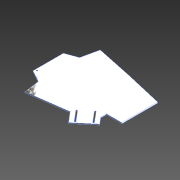
# Autodesk Inventor part: baseframe
Saved by Autodesk Inventor 2018 (Build 220112000, 112)
## iProperties
Created: 2018-05-27
Part Number: baseframe
Material: アルミニウム 6061
Document SubType Name: Sheet Metal
Designer: NaMACHAN
Mass: 118.519 g
Surface Area: 451.786 cm^2
Volume: 43.8959 cm^3
Density: 2.7 g/cm^3
Sheet Metal Rule: Default
Appearance: アルミニウム - フラット
Author: NaMACHAN
Autodesk Inventor part; units mm, degrees
ref_plane "YZ Plane" through (0, 0, 0) normal (1, 0, 0) x (0, 1, 0)
ref_plane "XZ Plane" through (0, 0, 0) normal (0, 1, 0) x (-1, 0, 0)
ref_plane "XY Plane" through (0, 0, 0) normal (0, 0, 1) x (1, 0, 0)
sketch "スケッチ1" plane through (0, 0, 0) normal (0, 0, 1) x (1, 0, 0)
  line L0 (-106.8804, 63.2098) -> (-114.8803, 63.2581) projected
  line L1 (-107.2922, -5.024) -> (-115.292, -4.9758) projected
  line L2 (-4.6996, 92.8548) -> (1.3002, 92.8186) projected
  line L3 (-5.3383, -12.9733) -> (0.6616, -13.0095) projected
  line L4 (-79.7382, 110.3105) -> (1.3027, 93.2276) projected
  line L5 (-88.2817, 72.7187) -> (-79.7382, 110.3105) projected
  line L6 (-84.055, -53.4485) -> (5.2045, -41.9275)
  line L7 (49.6711, -27.8017) -> (49.6711, -11.6868)
  line L8 (49.6711, -11.6868) -> (84.6711, -11.6868)
  line L9 (5.2045, -41.9275) -> (20.2045, -67.9083)
  line L10 (20.2045, -67.9083) -> (59.6711, -45.1223)
  line L11 (59.6711, -45.1223) -> (49.6711, -27.8017)
  line L12 (-84.055, -53.4485) -> (-90.292, -5.1266)
  circle A0 centre (-111.2619, 0) radius 1.5 projected
  circle A1 centre (-110.9105, 58.2341) radius 1.5 projected
  line L13 (-115.292, -4.9758) -> (-114.8803, 63.2581) projected
  line L14 (-106.8804, 63.2098) -> (-114.8803, 63.2581) projected
  line L15 (-106.8804, 63.2098) -> (-107.2922, -5.024) projected
  line L16 (-107.2922, -5.024) -> (-115.292, -4.9758) projected
  line L17 (-90.292, -5.1266) -> (-115.292, -4.9758)
  line L18 (-115.292, -4.9758) -> (-114.8803, 63.2581)
  circle A2 centre (-1.7299, 87.8368) radius 1.5 projected
  circle A3 centre (-2.3082, -7.9915) radius 1.5 projected
  line L19 (1.3002, 92.8186) -> (0.6616, -13.0095) projected
  line L20 (-5.3383, -12.9733) -> (0.6616, -13.0095) projected
  line L21 (-5.3383, -12.9733) -> (-4.6996, 92.8548) projected
  line L22 (-4.6996, 92.8548) -> (1.3002, 92.8186) projected
  line L23 (-114.8803, 63.2581) -> (-4.6996, 92.8548)
  line L24 (1.3002, 92.8186) -> (-4.6996, 92.8548)
  line L25 (1.3002, 92.8186) -> (35.0935, 58.6149)
  line L26 (35.0935, 58.6149) -> (85.0935, 58.3132)
  line L27 (85.0935, 58.3132) -> (84.6711, -11.6868)
  line L28 (-91.5437, -34.2492) -> (2.6068, -22.0969) projected
  point P0 (0, 0)
  dimension "d25" = 35
  dimension "d27" = 90
  dimension "d29" = 20
  dimension "d30" = 150
  dimension "d31" = 30
  dimension "d60" = 25
  dimension "d61" = 20
  dimension "d62" = 135
  dimension "d63" = 200
  dimension "d64" = 50
  dimension "d65" = 70
  constraints: 28 end point, 7 perpendicular, 2 parallel, 1 vertical
  measures "d25" distance of L7.end L8.end
  measures "d27" distance of L6.start L6.end
  measures "d29" distance of L10.end L7.start
  measures "d30" angle of L7 L11
  measures "d31" distance of L6.end L9.end
  measures "d60" horizontal distance of L12.end L13.start
  measures "d61" distance between parallel lines of L6 L28
  measures "d62" angle of L25 L26
  measures "d63" distance between parallel lines of L13 L27
  measures "d64" horizontal distance of L25.end L26.end
  measures "d65" vertical distance of L26.end L8.end
extrude "プレート2" add sketch "スケッチ1" along normal blind 2
equation "\"d6\" = Thickness"
equation "\"BendRadius\" = Thickness"
equation "\"BendReliefWidth\" = Thickness"
equation "\"BendReliefDepth\" = 0.5 * Thickness"
equation "\"CornerReliefSize\" = 4 * Thickness"
equation "\"MinimumRemnant\" = 2 * Thickness"
equation "\"TransitionRadius\" = BendRadius"
equation "\"JacobiRadiusSize\" = Thickness"
equation "\"GapSize\" = Thickness"
equation "\"Thickness\" = 2"
